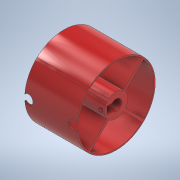
# Autodesk Inventor part: Rampa
Saved by Autodesk Inventor 2021 (Build 250183000, 183)
## iProperties
Created: 2022-11-24
Part Number: Rampa
Material: Genérico
Document SubType Name: Modeling
Designer: sergi
Density: 1 g/cm^3
Appearance: Valor por defecto
Author: sergi
Autodesk Inventor part; units mm, degrees
ref_plane "Plano de trabajo3" through (185, 53, 51.5) normal (1, 0, 0) x (0, 0, -1)
ref_plane "Plano de trabajo4" through (125.2094, 54.5, 50) normal (1, 0, 0) x (0, 0, -1)
sketch "Boceto3" plane through (125.2094, 54.5, 50) normal (1, 0, 0) x (0, 0, -1)
  circle A0 centre (0, 0) radius 30
  circle A1 centre (0, 0) radius 5
  point P0 (50, -54.5)
  dimension "d5" = 60
  dimension "d9" = 10
  constraints: 2 centre point, 1 coincident
  measures "d5" diameter of A0
  measures "d9" diameter of A1
extrude "Extrusión1" add sketch "Boceto3" along normal blind 40 contours A0 | A1
shell "Vaciado1" thickness 1 removed faces 2 at (125.2094, 56.8932, 44.7392) at (165.2094, 56.8932, 44.7392)
sketch "Boceto4" plane through (165.2094, 54.5, 50) normal (1, 0, 0) x (0, 0, -1)
  circle A0 centre (0, 0) radius 9
  circle A1 centre (0, 0) radius 4.1
  point P0 (50, -54.5)
  dimension "d10" = 18
  dimension "d11" = 8.2
  constraints: 2 centre point, 1 coincident
  measures "d10" diameter of A0
  measures "d11" diameter of A1
extrude "Extrusión2" add sketch "Boceto4" against normal blind 40
sketch "Boceto5" plane through (165.2094, 54.5, 50) normal (1, 0, 0) x (0, 0, -1)
  line L0 (0, 0) -> (-4.1, 0)
  circle A0 centre (0, 0) radius 4.1 projected
  line L1 (-4.1, 0) -> (-7.1, 0)
  line L2 (-1.1, -2.75) -> (-7.1, -2.75)
  line L3 (-7.1, -2.75) -> (-7.1, 2.75)
  line L4 (-7.1, 2.75) -> (-1.1, 2.75)
  line L5 (-1.1, 2.75) -> (-1.1, -2.75)
  line L6 (-1.1, -2.75) -> (-7.1, 2.75) construction
  line L7 (-7.1, -2.75) -> (-1.1, 2.75) construction
  point P0 (50, -54.5)
  point P1 (-3.041, -2.75)
  point P2 (-3.041, 2.75)
  dimension "d14" = 3
  dimension "d15" = 5.5
  constraints: 16 end point, 3 horizontal, 2 midpoint, 2 parallel, 1 perpendicular, 2 other
  measures "d14" distance of L0.end L1.end
  measures "d15" distance of L2.end L3.end
extrude "Extrusión3" cut sketch "Boceto5" against normal blind 5.5 contours L1 L3 L4 A0 | A0 L2 L3 L1
sketch "Boceto6" plane through (165.2094, 51.75, 57.1) normal (0, 0, -1) x (-1, 0, 0)
  line L0 (0, 0) -> (0, 5.5) projected
  line L1 (0, 0) -> (5.5, 0) projected
  line L2 (5.5, 0) -> (5.5, 5.5) projected
  line L3 (0, 5.5) -> (5.5, 5.5) projected
  line L4 (5.5, 0) -> (5.5, 5.5) projected
  line L5 (5.5, 5.5) -> (0, 0)
  circle A0 centre (2.75, 2.75) radius 1.5
  point P0 (165.2094, -51.75)
  dimension "d18" = 3
  constraints: 2 end point, 1 centre point, 1 midpoint
  measures "d18" diameter of A0
hole "Agujero1" at (162.4594, 54.5, 57.1) direction (0, 0, 1) diameter 3 depth 3.7 tip angle 118
ref_plane "Plano de trabajo5" through (145.2094, 54.5, 50) normal (1, 0, 0) x (0, 0, -1)
ref_plane "Plano de trabajo6" through (0, 0, 80) normal (0, 0, 1) x (1, 0, 0)
sketch "Boceto7" plane through (0, 0, 80) normal (0, 0, 1) x (1, 0, 0)
  line L0 (162.4594, 56) -> (162.4594, 53)
  circle A0 centre (162.4594, 54.5) radius 3.5
  point P0 (0, 0)
  dimension "d27" = 7
  constraints: 2 end point, 1 centre point, 1 midpoint, 1 vertical, 1 vertical alignment, 1 other
  measures "d27" diameter of A0
extrude "Extrusión4" cut sketch "Boceto7" against normal blind 5.5
mirror "Simetría2" about plane through (145.2094, 54.5, 50) normal (1, 0, 0) of "Extrusión4", "Agujero1", "Extrusión3"
sketch "Boceto10" plane through (165.2094, 54.5, 50) normal (1, 0, 0) x (0, 0, -1)
  line L0 (20.5061, -21.9203) -> (21.9203, -20.5061)
  line L1 (21.9203, -20.5061) -> (-20.5061, 21.9203)
  line L2 (-20.5061, 21.9203) -> (-21.9203, 20.5061)
  line L3 (-21.9203, 20.5061) -> (20.5061, -21.9203)
  line L4 (20.5061, -21.9203) -> (-20.5061, 21.9203) construction
  line L5 (21.9203, -20.5061) -> (-21.9203, 20.5061) construction
  line L6 (21.9203, 20.5061) -> (20.5061, 21.9203)
  line L7 (20.5061, 21.9203) -> (-21.9203, -20.5061)
  line L8 (-21.9203, -20.5061) -> (-20.5061, -21.9203)
  line L9 (-20.5061, -21.9203) -> (21.9203, 20.5061)
  line L10 (21.9203, 20.5061) -> (-21.9203, -20.5061) construction
  line L11 (20.5061, 21.9203) -> (-20.5061, -21.9203) construction
  line L12 (-3.041, -2.75) -> (-7.1, -2.75) projected
  line L13 (-7.1, -2.75) -> (-7.1, 2.75) projected
  line L14 (-7.1, 2.75) -> (-3.041, 2.75) projected
  arc A0 (-3.041, -2.75) -> (-3.041, 2.75) centre (0, 0) ccw projected
  circle A1 centre (0, 0) radius 9 projected
  circle A2 centre (0, 0) radius 9
  point P0 (50, -54.5)
  point P1 (0, 0)
  point P2 (2.1045, 3.5187)
  point P3 (3.5187, 2.1045)
  point P4 (-2.1045, -3.5187)
  point P5 (-4.1642, -2.75)
  point P6 (-4.1642, 2.75)
  point P7 (-2.1045, 3.5187)
  point P8 (3.5187, -2.1045)
  point P9 (2.1045, -3.5187)
  dimension "d30" = 2
  dimension "d31" = 60
  dimension "d32" = 2
  dimension "d33" = 60
  constraints: 24 end point, 4 midpoint, 4 parallel, 2 perpendicular, 1 centre point, 1 coincident, 1 concentric
  measures "d30" distance of L2.end L1.end
  measures "d31" distance of L1.end L0.end
  measures "d32" distance of L8.end L7.end
  measures "d33" distance of L7.end L6.end
extrude "Extrusión5" add sketch "Boceto10" against normal blind 40 contours L3 A1 L1 L0 | L3 A0 L1 A1 | A1 L7 L12 A0 L9 | L9 L8 L7 A1 | A0 L7 A1 L9 | A1 L7 L6 L9 | A1 L1 A0 L14 L3 | L3 L2 L1 A1
